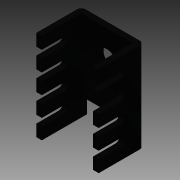
# Autodesk Inventor part: TO-220 Heatsink
Saved by Autodesk Inventor 2015 (Build 190159000, 159)
## iProperties
Created: 2016-01-19
Part Number: TO-220 Heatsink
Material: Generic
Document SubType Name: Modeling
Designer: Kyle
Density: 1 g/cm^3
Appearance: Anodized - Black
Author: Kyle
Autodesk Inventor part; units mm, degrees
ref_plane "YZ Plane" through (0, 0, 0) normal (1, 0, 0) x (0, 1, 0)
ref_plane "XZ Plane" through (0, 0, 0) normal (0, 1, 0) x (-1, 0, 0)
ref_plane "XY Plane" through (0, 0, 0) normal (0, 0, 1) x (1, 0, 0)
sketch "Sketch1" plane through (0, 0, 0) normal (0, 0, 1) x (1, 0, 0)
  line L0 (0, 0) -> (13.2105, 0)
  line L1 (13.2105, 0) -> (13.2105, 15.1511)
  line L2 (13.2105, 15.1511) -> (0, 15.1511)
  line L3 (0, 15.1511) -> (0, 0)
  circle A0 centre (6.6053, 9.431) radius 1.905
  dimension "d0" = 13.2105
  dimension "d1" = 15.1511
  dimension "d2" = 3.81
  dimension "d3" = 5.7201
  constraints: 8 end point, 2 parallel, 1 centre point, 1 horizontal, 1 perpendicular
  measures "d0" distance of L1.end L2.end
  measures "d1" distance of L0.end L1.end
  measures "d2" diameter of A0
  measures "d3" distance from line of L2 A0.centre
extrude "Extrusion1" add sketch "Sketch1" along normal blind 1.1989
sketch "Sketch2" plane through (0, 0, 0) normal (0, -1, 0) x (1, 0, 0)
  line L0 (0, 0) -> (13.2105, 0) projected
  line L1 (0, 1.1989) -> (1.1989, 1.1989)
  line L2 (1.1989, 1.1989) -> (1.1989, 0)
  line L3 (1.1989, 0) -> (0, 0)
  line L4 (0, 0) -> (0, 1.1989)
  line L5 (13.2105, 1.1989) -> (12.0117, 1.1989)
  line L6 (12.0117, 1.1989) -> (12.0117, 0)
  line L7 (12.0117, 0) -> (13.2105, 0)
  line L8 (13.2105, 0) -> (13.2105, 1.1989)
  dimension "d6" = 1.1989
  dimension "d7" = 1.1989
  constraints: 16 end point, 4 parallel, 2 horizontal, 2 perpendicular, 2 point on line
  measures "d6" distance of L1.start L1.end
  measures "d7" distance of L5.start L5.end
extrude "Extrusion2" add sketch "Sketch2" along normal blind 3.8989
sketch "Sketch3" plane through (0, 0, 1.1989) normal (0, 0, 1) x (1, 0, 0)
  line L0 (13.2105, -3.8989) -> (12.0117, -3.8989)
  line L1 (12.0117, -3.8989) -> (12.0117, 15.1511)
  line L2 (12.0117, 15.1511) -> (13.2105, 15.1511)
  line L3 (13.2105, 15.1511) -> (13.2105, -3.8989)
  line L4 (0, -3.8989) -> (1.1989, -3.8989)
  line L5 (1.1989, -3.8989) -> (1.1989, 15.1511)
  line L6 (1.1989, 15.1511) -> (0, 15.1511)
  line L7 (0, 15.1511) -> (0, -3.8989)
  point P0 (0, 0)
  constraints: 16 end point, 4 parallel, 2 horizontal, 2 perpendicular, 1 point on line
extrude "Extrusion3" add sketch "Sketch3" along normal blind 8.3312
sketch "Sketch4" plane through (13.2105, -3.8989, 0) normal (1, 0, 0) x (0, 0, -1)
  line L0 (-9.5301, 19.05) -> (-9.5301, 0) projected
  line L1 (0, 19.05) -> (-9.5301, 19.05) projected
  line L2 (0, 19.05) -> (0, 0) projected
  line L3 (-9.5301, 16.5506) -> (-4.0005, 16.5506)
  line L4 (-4.0005, 16.5506) -> (-4.0005, 14.8996)
  line L5 (-4.0005, 14.8996) -> (-9.5301, 14.8996)
  line L6 (-9.5301, 14.8996) -> (-9.5301, 16.5506)
  line L7 (-9.5301, 12.4003) -> (-4.0005, 12.4003)
  line L8 (-4.0005, 12.4003) -> (-4.0005, 10.7493)
  line L9 (-4.0005, 10.7493) -> (-9.5301, 10.7493)
  line L10 (-9.5301, 10.7493) -> (-9.5301, 12.4003)
  line L11 (-9.5301, 8.2499) -> (-4.0005, 8.2499)
  line L12 (-4.0005, 8.2499) -> (-4.0005, 6.5989)
  line L13 (-4.0005, 6.5989) -> (-9.5301, 6.5989)
  line L14 (-9.5301, 6.5989) -> (-9.5301, 8.2499)
  line L15 (-9.5301, 4.097) -> (-4.0005, 4.097)
  line L16 (-4.0005, 4.097) -> (-4.0005, 2.446)
  line L17 (-4.0005, 2.446) -> (-9.5301, 2.446)
  line L18 (-9.5301, 2.446) -> (-9.5301, 4.097)
  point P0 (0, 3.8989)
  point P1 (-9.5301, 2.446)
  point P2 (-4.0005, 19.05)
  dimension "d12" = 2.4994
  dimension "d13" = 1.651
  dimension "d14" = 2.4994
  dimension "d15" = 1.651
  dimension "d16" = 2.4994
  dimension "d17" = 1.651
  dimension "d18" = 2.5019
  dimension "d19" = 1.651
  dimension "d20" = 4.0005
  constraints: 32 end point, 8 parallel, 4 horizontal, 4 perpendicular, 4 point on line, 9 other
  measures "d12" distance from line of L3.start L1
  measures "d13" distance of point (-9.53, 14.9) L3.start
  measures "d14" distance of L7.start point (-9.53, 14.9)
  measures "d15" distance of point (-9.53, 10.749) L7.start
  measures "d16" distance of L11.start point (-9.53, 10.749)
  measures "d17" distance of point (-9.53, 6.599) L11.start
  measures "d18" distance of L15.start point (-9.53, 6.599)
  measures "d19" distance of point (-9.53, 2.446) L15.start
  measures "d20" distance from line of L2 point (-4.001, 19.05)
extrude "Extrusion4" cut sketch "Sketch4" against normal blind 25.4
fillet "Fillet1" radius 0.8255 16 edges at (12.6111, 11.0007, 4.0005) (12.6111, 6.8504, 4.0005) (12.6111, 2.7, 4.0005) (0.5994, -1.4529, 4.0005) (12.6111, -1.4529, 4.0005) (0.5994, 11.0007, 4.0005) (0.5994, 6.8504, 4.0005) (0.5994, 2.7, 4.0005) (12.6111, 12.6517, 4.0005) (12.6111, 8.5014, 4.0005) (12.6111, 4.351, 4.0005) (12.6111, 0.1981, 4.0005) (0.5994, 12.6517, 4.0005) (0.5994, 8.5014, 4.0005) (0.5994, 4.351, 4.0005) (0.5994, 0.1981, 4.0005)
fillet "Fillet2" radius 0.8255 2 edges at (13.2105, 5.6261, 0) (0, 5.6261, 0)
body "Solid1"
